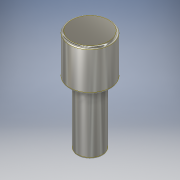
# Autodesk Inventor part: locatingpin
Saved by Autodesk Inventor 2017 (Build 210142000, 142)
## iProperties
Created: 2020-01-12
Part Number: locatingpin
Material: Silver
Document SubType Name: Modeling
Designer: Admin
Density: 10.49 g/cm^3
Appearance: Silver
Mass: 3.3016 g
Surface Area: 2.98189 cm^2
Volume: 0.314738 cm^3
Author: Admin
Autodesk Inventor part; units mm, degrees
ref_plane "YZ Plane" through (0, 0, 0) normal (1, 0, 0) x (0, 1, 0)
ref_plane "XZ Plane" through (0, 0, 0) normal (0, 1, 0) x (-1, 0, 0)
ref_plane "XY Plane" through (0, 0, 0) normal (0, 0, 1) x (1, 0, 0)
sketch "Sketch1" plane through (0, 0, 0) normal (0, 1, 0) x (-1, 0, 0)
  circle A0 centre (0, 0) radius 3.175
  circle A1 centre (0, 0) radius 1.9558
  dimension "d0" = 6.35
  dimension "d1" = 3.9116
  constraints: 2 centre point, 2 coincident
  measures "d0" diameter of A0
  measures "d1" diameter of A1
extrude "Extrusion1" add sketch "Sketch1" along normal blind 6.35 contours A0 | A1
extrude "Extrusion2" add sketch "Sketch1" against normal blind 9.525 contours A1
fillet "Fillet1" radius 0.3175 4 edges at (3.175, 6.35, 0) (1.9558, -9.525, 0) (3.175, 0, 0) (1.9558, 0, 0)
body "Solid1"
